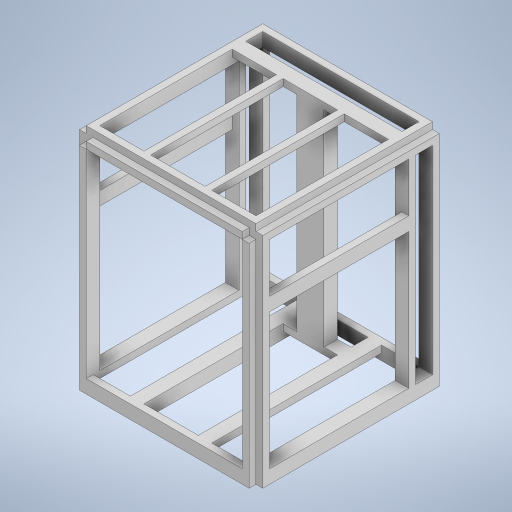
# Autodesk Inventor part: Rev V Envelope Frame Study
Saved by Autodesk Inventor 2024 (Build 280153000, 153)
## iProperties
Created: 2024-12-18
Part Number: Rev V Envelope Frame Study
Material: Generic
Document SubType Name: Modeling
Designer: Ishaan
Density: 1 g/cm^3
Appearance: Default
Author: Ishaan
Autodesk Inventor part; units mm, degrees
ref_plane "YZ Plane" through (0, 0, 0) normal (1, 0, 0) x (0, 1, 0)
ref_plane "XZ Plane" through (0, 0, 0) normal (0, 1, 0) x (-1, 0, 0)
ref_plane "XY Plane" through (0, 0, 0) normal (0, 0, 1) x (1, 0, 0)
sketch "Sketch10" plane through (0, 0, 0) normal (0, 1, 0) x (-1, 0, 0)
  line L0 (270, -270) -> (230, -270)
  line L1 (230, -270) -> (230, -230)
  line L2 (230, -230) -> (270, -230)
  line L3 (270, -230) -> (270, -270)
  line L4 (-230, 230) -> (-270, 230)
  line L5 (-270, 230) -> (-270, 270)
  line L6 (-270, 270) -> (-230, 270)
  line L7 (-230, 270) -> (-230, 230)
  line L8 (270, 230) -> (230, 230)
  line L9 (230, 230) -> (230, 270)
  line L10 (230, 270) -> (270, 270)
  line L11 (270, 270) -> (270, 230)
  line L12 (-230, 230) -> (230, 230) construction
  line L13 (230, 230) -> (230, -230) construction
  line L14 (230, -230) -> (-230, -230) construction
  line L15 (-230, -230) -> (-230, 230) construction
  line L16 (-230, 230) -> (230, -230) construction
  line L17 (230, 230) -> (-230, -230) construction
  line L18 (-230, -230) -> (-270, -230)
  line L19 (-270, -230) -> (-270, -270)
  line L20 (-270, -270) -> (-230, -270)
  line L21 (-230, -270) -> (-230, -230)
  line L22 (270, -270) -> (230, -270)
  line L23 (230, -270) -> (230, -250)
  line L24 (230, -250) -> (270, -250)
  line L25 (270, -250) -> (270, -270)
  line L26 (-270, -270) -> (-230, -270)
  line L27 (-230, -270) -> (-230, -250)
  line L28 (-230, -250) -> (-270, -250)
  line L29 (-270, -250) -> (-270, -270)
  line L30 (-270, 270) -> (-250, 270)
  line L31 (-250, 270) -> (-250, 250)
  line L32 (-250, 250) -> (-270, 250)
  line L33 (-270, 250) -> (-270, 270)
  line L34 (270, 270) -> (250, 270)
  line L35 (250, 270) -> (250, 250)
  line L36 (250, 250) -> (270, 250)
  line L37 (270, 250) -> (270, 270)
  point P0 (0, 0)
  point P1 (230, -270)
  point P2 (-250, 270)
  point P3 (-230, -250)
  point P4 (230, -250)
  dimension "d71" = 40
  dimension "d72" = 40
  dimension "d75" = 40
  dimension "d76" = 40
  dimension "d77" = 40
  dimension "d78" = 40
  dimension "d79" = 460
  dimension "d80" = 460
  dimension "d81" = 40
  dimension "d82" = 40
  dimension "d83" = 40
  dimension "d84" = 20
  dimension "d85" = 40
  dimension "d86" = 20
  dimension "d87" = 20
  dimension "d88" = 20
  dimension "d89" = 20
  dimension "d90" = 20
  constraints: 76 end point, 18 parallel, 9 horizontal, 9 perpendicular, 2 midpoint, 1 point on line
  measures "d71" distance of L1.end L2.end
  measures "d72" distance of L1.end L0.end
  measures "d75" distance of L5.end L6.end
  measures "d76" distance of L4.end L5.end
  measures "d77" distance of L9.end L10.end
  measures "d78" distance of L8.end L9.end
  measures "d79" distance of L1.end L14.end
  measures "d80" distance of L8.end L1.end
  measures "d81" distance of L20.end L19.end
  measures "d82" distance of L19.end L18.end
  measures "d83" distance of L23.end L24.end
  measures "d84" distance of L22.end L23.end
  measures "d85" distance of L28.end L27.end
  measures "d86" distance of L27.end L26.end
  measures "d87" distance of L31.end L32.end
  measures "d88" distance of L30.end L31.end
  measures "d89" distance of L36.end L35.end
  measures "d90" distance of L35.end L34.end
extrude "Extrusion10" add sketch "Sketch10" along normal blind 625 contours L0 L1 L24 L3 | L4 L5 L32 L31 L6 L7 | L8 L9 L10 L35 L36 L11 | L21 L20 L19 L28
sketch "Sketch11" plane through (-270, 0, 250) normal (0, 0, 1) x (1, 0, 0)
  line L0 (0, 0) -> (20, 0) projected
  line L1 (20, 0) -> (20, 625) projected
  line L2 (0, 625) -> (20, 625) projected
  line L3 (0, 0) -> (0, 625) projected
  line L4 (520, 0) -> (540, 0) projected
  line L5 (540, 0) -> (540, 625) projected
  line L6 (520, 625) -> (540, 625) projected
  line L7 (520, 0) -> (520, 625) projected
  line L8 (540, 625) -> (500, 625)
  line L9 (500, 625) -> (500, 665)
  line L10 (500, 665) -> (540, 665)
  line L11 (540, 665) -> (540, 625)
  line L12 (0, 625) -> (40, 625)
  line L13 (40, 625) -> (40, 665)
  line L14 (40, 665) -> (0, 665)
  line L15 (0, 665) -> (0, 625)
  line L16 (0, 665) -> (20, 665)
  line L17 (20, 665) -> (20, 645)
  line L18 (20, 645) -> (0, 645)
  line L19 (0, 645) -> (0, 665)
  line L20 (540, 665) -> (520, 665)
  line L21 (520, 665) -> (520, 645)
  line L22 (520, 645) -> (540, 645)
  line L23 (540, 645) -> (540, 665)
  point P0 (270, 0)
  point P1 (0, 645)
  point P2 (20, 625)
  dimension "d93" = 40
  dimension "d94" = 40
  dimension "d95" = 40
  dimension "d96" = 40
  dimension "d97" = 20
  dimension "d98" = 20
  dimension "d99" = 20
  dimension "d100" = 20
  constraints: 32 end point, 8 parallel, 4 horizontal, 4 perpendicular
  measures "d93" distance of L9.end L10.end
  measures "d94" distance of L8.end L9.end
  measures "d95" distance of L14.end L13.end
  measures "d96" distance of L13.end L12.end
  measures "d97" distance of L17.end L18.end
  measures "d98" distance of L16.end L17.end
  measures "d99" distance of L22.end L21.end
  measures "d100" distance of L21.end L20.end
extrude "Extrusion11" add sketch "Sketch11" against normal up to surface (520 mm away) separate body contours L15 L18 L17 L14 L13 L12 L2 | L8 L9 L10 L21 L22 L11 L6
sketch "Sketch12" plane through (-230, 625, 250) normal (1, 0, 0) x (0, 0, -1)
  line L0 (520, 0) -> (520, 40) projected
  line L1 (0, 40) -> (520, 40) projected
  line L2 (0, 0) -> (0, 40) projected
  line L3 (0, 0) -> (520, 0) projected
  line L4 (20, 40) -> (-20, 40)
  line L5 (-20, 40) -> (-20, 0)
  line L6 (-20, 0) -> (20, 0)
  line L7 (20, 0) -> (20, 40)
  line L8 (-20, 40) -> (0, 40)
  line L9 (0, 40) -> (0, 20)
  line L10 (0, 20) -> (-20, 20)
  line L11 (-20, 20) -> (-20, 40)
  line L12 (500, 40) -> (520, 40)
  line L13 (520, 40) -> (520, 0)
  line L14 (520, 0) -> (500, 0)
  line L15 (500, 0) -> (500, 40)
  point P0 (250, -625)
  point P1 (20, 0)
  point P2 (20, 40)
  point P3 (500, 40)
  point P4 (500, 0)
  dimension "d103" = 40
  dimension "d104" = 40
  dimension "d105" = 20
  dimension "d106" = 20
  dimension "d107" = 20
  dimension "d108" = 40
  constraints: 24 end point, 6 parallel, 3 horizontal, 3 perpendicular
  measures "d103" distance of L6.end L5.end
  measures "d104" distance of L5.end L4.end
  measures "d105" distance of L9.end L10.end
  measures "d106" distance of L1.start L9.end
  measures "d107" distance of L13.end L14.end
  measures "d108" distance of L0.end L13.end
extrude "Extrusion12" add sketch "Sketch12" along normal up to surface (460 mm away) separate body contours L3 L15 L1 L0 | L3 L2 L1 L7 | L6 L5 L10 L2
sketch "Sketch13" plane through (-270, 0, -250) normal (0, 0, 1) x (1, 0, 0)
  line L0 (540, 0) -> (500, 0)
  line L1 (500, 0) -> (500, 40)
  line L2 (500, 40) -> (540, 40)
  line L3 (540, 40) -> (540, 0)
  line L4 (0, 0) -> (40, 0)
  line L5 (40, 0) -> (40, 40)
  line L6 (40, 40) -> (0, 40)
  line L7 (0, 40) -> (0, 0)
  line L8 (40, 0) -> (0, 0) projected
  line L9 (0, 0) -> (0, 625) projected
  line L10 (0, 625) -> (40, 625) projected
  line L11 (40, 625) -> (40, 0) projected
  line L12 (540, 0) -> (500, 0) projected
  line L13 (500, 0) -> (500, 625) projected
  line L14 (500, 625) -> (540, 625) projected
  line L15 (540, 625) -> (540, 0) projected
  line L16 (500, 665) -> (520, 665) projected
  line L17 (520, 665) -> (520, 645) projected
  line L18 (520, 645) -> (540, 645) projected
  line L19 (540, 645) -> (540, 625) projected
  line L20 (500, 625) -> (500, 665) projected
  line L21 (0, 625) -> (0, 645) projected
  line L22 (0, 645) -> (20, 645) projected
  line L23 (20, 645) -> (20, 665) projected
  line L24 (20, 665) -> (40, 665) projected
  line L25 (40, 665) -> (40, 625) projected
  line L26 (40, 625) -> (0, 625) projected
  line L27 (500, 625) -> (40, 625) projected
  line L28 (40, 625) -> (40, 665) projected
  line L29 (40, 665) -> (500, 665) projected
  line L30 (500, 665) -> (500, 625) projected
  line L31 (540, 625) -> (500, 625) projected
  line L32 (500, 0) -> (500, 625) projected
  line L33 (500, 0) -> (520, 0)
  line L34 (520, 0) -> (520, 20)
  line L35 (520, 20) -> (500, 20)
  line L36 (500, 20) -> (500, 0)
  line L37 (40, 0) -> (20, 0)
  line L38 (20, 0) -> (20, 20)
  line L39 (20, 20) -> (40, 20)
  line L40 (40, 20) -> (40, 0)
  point P0 (270, 0)
  point P1 (520, 0)
  dimension "d113" = 40
  dimension "d114" = 40
  dimension "d115" = 40
  dimension "d116" = 40
  dimension "d212" = 20
  dimension "d213" = 20
  dimension "d214" = 20
  dimension "d215" = 20
  constraints: 32 end point, 8 parallel, 4 horizontal, 4 perpendicular
  measures "d113" distance of L1.end L2.end
  measures "d114" distance of L0.end L1.end
  measures "d115" distance of L6.end L5.end
  measures "d116" distance of L4.end L5.end
  measures "d212" distance of L35.end L34.end
  measures "d213" distance of L34.end L33.end
  measures "d214" distance of L38.end L39.end
  measures "d215" distance of L37.end L38.end
extrude "Extrusion13" add sketch "Sketch13" along normal up to surface (480 mm away) separate body contours L0 L34 L35 L1 L2 L3 | L5 L39 L38 L4 L7 L6
sketch "Sketch14" plane through (-230, 0, 270) normal (1, 0, 0) x (0, 0, -1)
  line L0 (0, 0) -> (40, 0) projected
  line L1 (40, 0) -> (40, 625) projected
  line L2 (0, 625) -> (40, 625) projected
  line L3 (0, 0) -> (0, 625) projected
  line L4 (520, 0) -> (540, 0) projected
  line L5 (540, 0) -> (540, 625) projected
  line L6 (520, 625) -> (540, 625) projected
  line L7 (520, 0) -> (520, 625) projected
  line L8 (0, 0) -> (20, 0)
  line L9 (20, 0) -> (20, 40)
  line L10 (20, 40) -> (0, 40)
  line L11 (0, 40) -> (0, 0)
  line L12 (540, 0) -> (520, 0)
  line L13 (520, 0) -> (520, 40)
  line L14 (520, 40) -> (540, 40)
  line L15 (540, 40) -> (540, 0)
  dimension "d216" = 20
  dimension "d217" = 40
  dimension "d218" = 20
  dimension "d219" = 40
  constraints: 16 end point, 4 parallel, 2 horizontal, 2 perpendicular
  measures "d216" distance of L10.end L9.end
  measures "d217" distance of L9.end L8.end
  measures "d218" distance of L13.end L14.end
  measures "d219" distance of L12.end L13.end
extrude "Extrusion14" add sketch "Sketch14" along normal up to surface (460 mm away) separate body contours L3 L10 L9 L0 | L7 L14 L5 L4
sketch "Sketch17" plane through (230, 40, -250) normal (0, 1, 0) x (1, 0, 0)
  line L0 (-460, -480) -> (-500, -480) projected
  line L1 (-460, 0) -> (-500, 0) projected
  line L2 (-460, 0) -> (-460, -480) projected
  line L3 (-500, 0) -> (-500, -480) projected
  line L4 (-500, -70) -> (-460, -70)
  line L5 (-460, -70) -> (-460, -50)
  line L6 (-460, -50) -> (-500, -50)
  line L7 (-500, -50) -> (-500, -70)
  line L8 (0, -70) -> (40, -70)
  line L9 (40, -70) -> (40, -50)
  line L10 (40, -50) -> (0, -50)
  line L11 (0, -50) -> (0, -70)
  line L12 (0, 0) -> (0, -480) projected
  line L13 (40, 0) -> (40, -480) projected
  point P0 (-230, -250)
  point P1 (-460, -50)
  point P2 (-500, -50)
  point P3 (-460, -70)
  dimension "d188" = 40
  dimension "d189" = 20
  dimension "d190" = 40
  dimension "d191" = 20
  dimension "d192" = 410
  constraints: 16 end point, 4 parallel, 2 collinear, 2 horizontal, 2 perpendicular, 1 point on line
  measures "d188" distance of L6.end L5.end
  measures "d189" distance of L5.end L4.end
  measures "d190" distance of L10.end L9.end
  measures "d191" distance of L9.end L8.end
  measures "d192" distance from line of L0.start L4
extrude "Extrusion17" add sketch "Sketch17" along normal up to surface (585 mm away) separate body contours L4 L3 L6 L2 | L11 L10 L9 L8
sketch "Sketch27" plane through (-230, 0, -250) normal (0, 0, 1) x (1, 0, 0)
  line L0 (460, 665) -> (480, 665) projected
  line L1 (480, 665) -> (480, 645) projected
  line L2 (480, 645) -> (500, 645) projected
  line L3 (500, 645) -> (500, 625) projected
  line L4 (460, 625) -> (460, 665) projected
  line L5 (-40, 625) -> (-40, 645) projected
  line L6 (-40, 645) -> (-20, 645) projected
  line L7 (-20, 645) -> (-20, 665) projected
  line L8 (-20, 665) -> (0, 665) projected
  line L9 (0, 665) -> (0, 625) projected
  line L10 (0, 625) -> (-40, 625) projected
  line L11 (330, 0) -> (130, 0)
  line L12 (130, 0) -> (130, 40)
  line L13 (130, 40) -> (330, 40)
  line L14 (330, 40) -> (330, 0)
  line L15 (330, 0) -> (130, 40) construction
  line L16 (130, 0) -> (330, 40) construction
  line L17 (310, 0) -> (150, 0)
  line L18 (150, 0) -> (150, 40)
  line L19 (150, 40) -> (310, 40)
  line L20 (310, 40) -> (310, 0)
  line L21 (310, 0) -> (150, 40) construction
  line L22 (150, 0) -> (310, 40) construction
  line L23 (500, 625) -> (460, 625) projected
  line L24 (-40, 40) -> (0, 40) projected
  line L25 (0, 40) -> (0, 20) projected
  line L26 (0, 20) -> (-20, 20) projected
  line L27 (-20, 20) -> (-20, 0) projected
  line L28 (-20, 0) -> (-40, 0) projected
  line L29 (-40, 0) -> (-40, 40) projected
  line L30 (480, 0) -> (480, 20) projected
  line L31 (480, 20) -> (460, 20) projected
  line L32 (460, 20) -> (460, 40) projected
  line L33 (500, 0) -> (480, 0) projected
  line L34 (460, 0) -> (0, 0) projected
  line L35 (0, 0) -> (0, 40) projected
  line L36 (0, 40) -> (460, 40) projected
  line L37 (0, 0) -> (-40, 0) projected
  line L38 (-40, 0) -> (-40, 625) projected
  line L39 (-40, 625) -> (0, 625) projected
  line L40 (0, 625) -> (0, 0) projected
  line L41 (460, 0) -> (460, 625) projected
  line L42 (460, 625) -> (500, 625) projected
  line L43 (500, 625) -> (500, 0) projected
  line L44 (460, 625) -> (0, 625) projected
  line L45 (0, 625) -> (0, 665) projected
  line L46 (0, 665) -> (460, 665) projected
  line L47 (460, 665) -> (460, 625) projected
  line L48 (150, 40) -> (110, 40)
  line L49 (110, 40) -> (110, 20)
  line L50 (110, 20) -> (150, 20)
  line L51 (150, 20) -> (150, 40)
  line L52 (310, 40) -> (350, 40)
  line L53 (350, 40) -> (350, 20)
  line L54 (350, 20) -> (310, 20)
  line L55 (310, 20) -> (310, 40)
  line L56 (460, 40) -> (500, 40) projected
  line L57 (500, 40) -> (500, 0) projected
  line L58 (460, 40) -> (460, 0) projected
  line L59 (500, 0) -> (460, 0) projected
  point P0 (230, 0)
  point P1 (230, 20)
  point P2 (230, 20)
  point P3 (150, 20)
  point P4 (310, 0)
  point P5 (150, 0)
  point P6 (330, 20)
  point P7 (350, 40)
  point P8 (130, 20)
  point P9 (110, 40)
  dimension "d194" = 20
  dimension "d195" = 160
  dimension "d220" = 40
  dimension "d221" = 20
  dimension "d222" = 40
  dimension "d223" = 20
  constraints: 40 end point, 8 parallel, 6 midpoint, 4 horizontal, 4 perpendicular, 2 collinear, 1 point on line, 1 vertical alignment, 1 other
  measures "d194" distance from line of point (150, 20) L12
  measures "d195" distance between parallel lines of L18 L20
  measures "d220" distance of L50.end L49.end
  measures "d221" distance of L49.end L48.end
  measures "d222" distance of L53.end L54.end
  measures "d223" distance of L52.end L53.end
extrude "Extrusion27" add sketch "Sketch27" along normal up to surface (500 mm away) separate body contours L53 L54 L14 L36 | L14 L54 L20 L13 | L36 L12 L50 L49 | L11 L20 L54 L14 | L13 L18 L50 L12 | L12 L50 L18 L11
sketch "Sketch32" plane through (-80, 0, -250) normal (1, 0, 0) x (0, 0, -1)
  line L0 (-70, 625) -> (-50, 625) projected
  line L1 (-70, 40) -> (-70, 625) projected
  line L2 (-70, 40) -> (-50, 40) projected
  line L3 (-50, 40) -> (-50, 625) projected
  line L4 (-50, 40) -> (-90, 40)
  line L5 (-90, 40) -> (-90, 20)
  line L6 (-90, 20) -> (-50, 20)
  line L7 (-50, 20) -> (-50, 40)
  point P0 (-250, 0)
  dimension "d224" = 40
  dimension "d225" = 20
  constraints: 8 end point, 2 parallel, 1 horizontal, 1 perpendicular
  measures "d224" distance of L6.end L5.end
  measures "d225" distance of L5.end L4.end
extrude "Extrusion31" add sketch "Sketch32" along normal up to surface (160 mm away) separate body contours L2 L7 L6 L5 L4
sketch "Sketch29" plane through (230, 625, 250) normal (-1, 0, 0) x (0, 0, 1)
  line L0 (-450, -585) -> (-450, 0) projected
  line L1 (0, 40) -> (-520, 40) projected
  line L2 (-450, 40) -> (-410, 40)
  line L3 (-410, 40) -> (-410, 20)
  line L4 (-410, 20) -> (-450, 20)
  line L5 (-450, 20) -> (-450, 40)
  point P0 (-250, -625)
  point P1 (-410, 40)
  dimension "d228" = 40
  dimension "d229" = 20
  constraints: 8 end point, 2 parallel, 1 collinear, 1 horizontal, 1 perpendicular, 1 point on line
  measures "d228" distance of L3.end L4.end
  measures "d229" distance of L2.end L3.end
extrude "Extrusion29" add sketch "Sketch29" along normal up to surface (460 mm away) separate body
sketch "Sketch30" plane through (-70, 40, -160) normal (0, 1, 0) x (1, 0, 0)
  line L0 (110, 40) -> (30, 40)
  line L1 (30, 40) -> (30, 0)
  line L2 (30, 0) -> (110, 0)
  line L3 (110, 0) -> (110, 40)
  line L4 (110, 40) -> (30, 0) construction
  line L5 (30, 40) -> (110, 0) construction
  line L6 (-10, 40) -> (150, 40) projected
  point P0 (70, -155)
  point P1 (70, 20)
  point P2 (70, 40)
  dimension "d208" = 80
  dimension "d209" = 40
  constraints: 12 end point, 4 midpoint, 2 parallel, 1 horizontal, 1 perpendicular
  measures "d208" distance of L2.end L1.end
  measures "d209" distance of L1.end L0.end
extrude "Extrusion30" add sketch "Sketch30" along normal up to surface (605 mm away) separate body
sketch "Sketch33" plane through (-230, 625, 230) normal (0, 0, -1) x (-1, 0, 0)
  line L0 (0, 20) -> (0, 40) projected
  line L1 (-460, 20) -> (0, 20) projected
  line L2 (-460, 20) -> (-460, 40) projected
  line L3 (-460, 40) -> (0, 40) projected
  line L4 (-310, 40) -> (-330, 40)
  line L5 (-330, 40) -> (-330, 20)
  line L6 (-330, 20) -> (-310, 20)
  line L7 (-310, 20) -> (-310, 40)
  line L8 (-150, 40) -> (-130, 40)
  line L9 (-130, 40) -> (-130, 20)
  line L10 (-130, 20) -> (-150, 20)
  line L11 (-150, 20) -> (-150, 40)
  point P0 (-230, -625)
  point P1 (-310, -585)
  point P2 (-150, -585)
  point P3 (-150, 20)
  point P4 (-130, 20)
  point P5 (-130, 40)
  point P6 (-310, 20)
  point P7 (-330, 40)
  point P8 (-330, 20)
  dimension "d230" = 20
  dimension "d231" = 20
  dimension "d232" = 20
  dimension "d233" = 20
  constraints: 16 end point, 4 parallel, 4 point on line, 2 horizontal, 2 perpendicular
  measures "d230" distance of L6.end L5.end
  measures "d231" distance of L5.end L4.end
  measures "d232" distance of L9.end L10.end
  measures "d233" distance of L8.end L9.end
extrude "Extrusion32" add sketch "Sketch33" along normal up to surface (390 mm away) separate body contours L1 L11 L3 L9 | L1 L5 L3 L7
sketch "Sketch34" plane through (270, 0, 230) normal (0, 0, -1) x (-1, 0, 0)
  line L0 (40, 0) -> (0, 0) construction
  line L1 (0, 0) -> (0, 625) construction
  line L2 (0, 625) -> (40, 625) construction
  line L3 (40, 625) -> (40, 0) construction
  line L4 (540, 625) -> (540, 0) construction
  line L5 (540, 0) -> (500, 0) construction
  line L6 (500, 0) -> (500, 625) construction
  line L7 (500, 625) -> (540, 625) construction
  line L8 (20, 665) -> (40, 665) construction
  line L9 (40, 665) -> (40, 625) construction
  line L10 (40, 625) -> (0, 625) construction
  line L11 (0, 625) -> (0, 645) construction
  line L12 (0, 645) -> (20, 645) construction
  line L13 (20, 645) -> (20, 665) construction
  line L14 (540, 645) -> (540, 625) construction
  line L15 (540, 625) -> (500, 625) construction
  line L16 (500, 625) -> (500, 665) construction
  line L17 (500, 665) -> (520, 665) construction
  line L18 (520, 665) -> (520, 645) construction
  line L19 (520, 645) -> (540, 645) construction
  line L20 (500, 665) -> (500, 625) construction
  line L21 (500, 625) -> (40, 625) construction
  line L22 (40, 625) -> (40, 665) construction
  line L23 (40, 665) -> (500, 665) construction
  line L24 (500, 40) -> (540, 40) construction
  line L25 (540, 40) -> (540, 0) construction
  line L26 (540, 0) -> (520, 0) construction
  line L27 (520, 0) -> (520, 20) construction
  line L28 (520, 20) -> (500, 20) construction
  line L29 (500, 20) -> (500, 40) construction
  line L30 (40, 20) -> (20, 20) construction
  line L31 (20, 20) -> (20, 0) construction
  line L32 (20, 0) -> (0, 0) construction
  line L33 (0, 0) -> (0, 40) construction
  line L34 (0, 40) -> (40, 40) construction
  line L35 (40, 40) -> (40, 20) construction
  line L36 (190, 40) -> (190, 0) construction
  line L37 (190, 0) -> (170, 0) construction
  line L38 (170, 0) -> (170, 20) construction
  line L39 (170, 20) -> (150, 20) construction
  line L40 (150, 20) -> (150, 40) construction
  line L41 (150, 40) -> (190, 40) construction
  line L42 (350, 40) -> (390, 40) construction
  line L43 (390, 40) -> (390, 20) construction
  line L44 (390, 20) -> (370, 20) construction
  line L45 (370, 20) -> (370, 0) construction
  line L46 (370, 0) -> (350, 0) construction
  line L47 (350, 0) -> (350, 40) construction
  line L48 (370, 645) -> (350, 645) construction
  line L49 (350, 645) -> (350, 665) construction
  line L50 (350, 665) -> (370, 665) construction
  line L51 (370, 665) -> (370, 645) construction
  line L52 (170, 665) -> (190, 665) construction
  line L53 (190, 665) -> (190, 645) construction
  line L54 (190, 645) -> (170, 645) construction
  line L55 (170, 645) -> (170, 665) construction
  line L56 (0, 40) -> (0, 625) construction
  line L57 (20, 0) -> (20, 625) construction
  line L58 (0, 480) -> (20, 480)
  line L59 (20, 480) -> (20, 440)
  line L60 (20, 440) -> (0, 440)
  line L61 (0, 440) -> (0, 480)
  point P0 (270, 0)
  dimension "d236" = 20
  dimension "d237" = 40
  dimension "d240" = 400
  constraints: 10 end point, 3 parallel, 1 collinear, 1 horizontal, 1 perpendicular
  measures "d236" distance of L59.end L60.end
  measures "d237" distance of L58.end L59.end
  measures "d240" distance between parallel lines of L34 L60
extrude "Extrusion33" add sketch "Sketch34" along normal up to surface (410 mm away) separate body
mirror "Mirror1" about plane through (0, 0, 0) normal (1, 0, 0) of "Extrusion33" bodies 12
combine bodies "Combine1" operation type add bodies to combine 2 3 4 5 6 7 9 10 8 11 12 1
equation "\"d80\" = d79"
body "Solid1"
body "Solid10"
